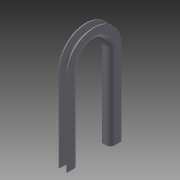
# Autodesk Inventor part: Filament Guide
Saved by Autodesk Inventor 2015 (Build 190159000, 159)
## iProperties
Created: 2014-08-31
Part Number: Filament Guide
Material: Generic
Document SubType Name: Modeling
Designer: Chris
Density: 1 g/cm^3
Appearance: Default
Author: Chris
Autodesk Inventor part; units mm, degrees
ref_plane "YZ Plane" through (0, 0, 0) normal (1, 0, 0) x (0, 1, 0)
ref_plane "XZ Plane" through (0, 0, 0) normal (0, 1, 0) x (-1, 0, 0)
ref_plane "XY Plane" through (0, 0, 0) normal (0, 0, 1) x (1, 0, 0)
sketch "Sketch3" plane through (0, 0, 0) normal (0, 0, 1) x (1, 0, 0)
  arc A0 (4, 0) -> (-4, 0) centre (0, 0) ccw
  line L0 (5, -0.9717) -> (5, -6.9717)
  line L1 (-5, -6.9717) -> (-5, 0)
  line L2 (-4, 0) -> (-4, -6.9717)
  line L3 (4, 0) -> (4, -6.9717)
  line L4 (5, -6.9717) -> (4, -6.9717)
  line L5 (-4, -6.9717) -> (-5, -6.9717)
  line L6 (-5, 0) -> (-5, 6)
  line L7 (-5, 6) -> (5, 6)
  line L8 (5, 6) -> (5, -0.9717)
  dimension "d9" = 8
  dimension "d11" = 6
  dimension "d29" = 10
  dimension "d30" = 6
  constraints: 18 end point, 4 perpendicular, 2 parallel, 2 point on circle, 2 tangent, 1 centre point, 1 coincident
  measures "d9" diameter of A0
  measures "d11" distance of L0.start L0.end
  measures "d29" distance of L6.end L7.end
  measures "d30" distance of L1.end L6.end
sketch "Sketch17" plane through (0, 0, 0) normal (1, 0, 0) x (0, 1, 0)
  line L0 (0, 0) -> (0, 100)
  line L1 (50, 100) -> (50, 0)
  arc A0 (50, 100) -> (0, 100) centre (25, 100) ccw
  dimension "d49" = 100
  dimension "d50" = 50
  dimension "d51" = 50
  constraints: 4 end point, 2 point on circle, 2 vertical, 1 centre point
  measures "d49" distance of L0.start L0.end
  measures "d50" distance of L0.end L1.start
  measures "d51" diameter of A0
sweep "Sweep1" add profiles "Sketch3" path "Sketch17"
fillet "Fillet6" radius 5 3 edges at (5, 6, 50) (5, 25, 119) (5, 44, 50)
body "Solid3"
